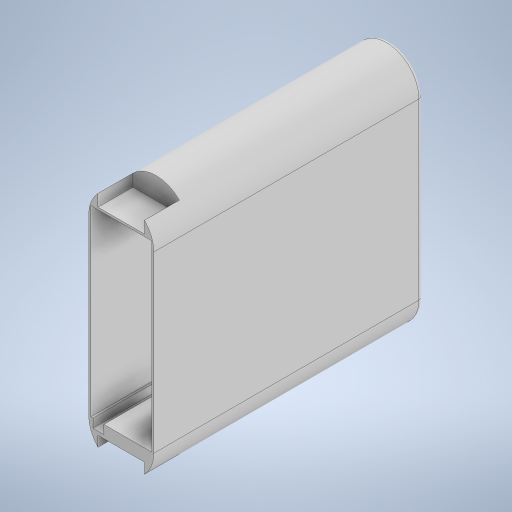
# Autodesk Inventor part: Carcasa Luis
Saved by Autodesk Inventor 2023.4 (Build 274418000, 418)
## iProperties
Created: 2024-01-25
Part Number: Carcasa Luis
Material: Genérico
Document SubType Name: Modeling
Designer: Adrián Álvarez
Density: 1 g/cm^3
Appearance: Valor por defecto
Author: Adrián Álvarez
Autodesk Inventor part; units mm, degrees
ref_plane "YZ Plane" through (0, 0, 0) normal (1, 0, 0) x (0, 1, 0)
ref_plane "XZ Plane" through (0, 0, 0) normal (0, 1, 0) x (-1, 0, 0)
ref_plane "XY Plane" through (0, 0, 0) normal (0, 0, 1) x (1, 0, 0)
sketch "Boceto1" plane through (0, 0, 0) normal (0, 0, 1) x (1, 0, 0)
  line L0 (0, 0) -> (0, 40.1) construction
  line L1 (7.5, 0) -> (7.5, 40.1)
  line L2 (-7.5, 40.1) -> (-7.5, 0)
  arc A0 (-7.5, 0) -> (7.5, 0) centre (0, 0) ccw
  arc A1 (7.5, 40.1) -> (-7.5, 40.1) centre (0, 40.1) ccw
  point P0 (0, 20.05)
  dimension "d0" = 40.1
  dimension "d1" = 15
  constraints: 8 end point, 4 point on circle, 4 tangent, 2 centre point, 1 midpoint, 1 parallel, 1 vertical
  measures "d0" distance of L0.start L0.end
  measures "d1" diameter of A1
extrude "Extrusión1" add sketch "Boceto1" along normal blind 62
sketch "Boceto2" plane through (0, 0, 62) normal (0, 0, 1) x (1, 0, 0)
  line L0 (0, 0) -> (-7, 0)
  line L1 (-7, 0) -> (-7, 40.0875)
  line L2 (-7.5, 40.1) -> (-7.5, 0) projected
  line L3 (7, 0) -> (-7, 0)
  line L4 (-7, 40.0875) -> (-7, 42.1)
  arc A0 (7.5, 40.1) -> (-7.5, 40.1) centre (0, 40.1) ccw projected
  line L5 (-7, 42.1) -> (7, 42.1)
  line L6 (7, 42.1) -> (7, 0)
  dimension "d4" = 7
  dimension "d68" = 7
  dimension "d69" = 14
  constraints: 12 end point, 2 horizontal, 1 parallel, 1 perpendicular, 1 vertical
  measures "d4" distance of L0.start L0.end
  measures "d68" distance of L3.start L0.start
  measures "d69" distance of L4.end L5.end
extrude "Extrusión2" cut sketch "Boceto2" against normal blind 61
sketch "Boceto3" plane through (0, 0, 62) normal (0, 0, 1) x (1, 0, 0)
  line L0 (-5.3571, -2.8499) -> (5.3571, -2.8499)
  line L1 (-6.5, 40.1) -> (6.5, 40.1) projected
  line L2 (-5, 42.6) -> (5, 42.6)
  line L3 (-5.3571, -2.8499) -> (-5.3571, -4.1499)
  line L4 (5.3571, -5.2489) -> (5.3571, -2.8499)
  arc A0 (7.5, 40.1) -> (-7.5, 40.1) centre (0, 40.1) ccw projected
  arc A1 (-5.3571, -5.2489) -> (5.3571, -5.2489) centre (0, 0) ccw
  line L5 (-5.3571, -4.1499) -> (-5.3571, -5.2489)
  arc A2 (-7.5, 0) -> (7.5, 0) centre (0, 0) ccw projected
  arc A3 (5.357, 45.3491) -> (-5.357, 45.3491) centre (0, 40.1) ccw
  line L6 (0, 42.6) -> (-5.357, 42.6)
  line L7 (-5.357, 42.6) -> (-5.357, 45.3491)
  line L8 (0, 42.6) -> (5.357, 42.6)
  line L9 (5.357, 42.6) -> (5.357, 45.3491)
  line L10 (0, -2.8499) -> (-5.357, -2.8499)
  point P0 (5.3571, -4.1499)
  point P1 (5, 43.9)
  dimension "d46" = 1.3
  dimension "d70" = 5.357
  dimension "d71" = 5.357
  dimension "d72" = 5.357
  constraints: 20 end point, 5 point on circle, 4 point on line, 2 centre point, 2 coincident, 2 midpoint, 2 perpendicular, 2 vertical
  measures "d46" distance of L0.start L3.end
  measures "d70" distance of L6.start L6.end
  measures "d71" distance of L6.start L8.end
  measures "d72" distance of L10.start L10.end
extrude "Extrusión3" cut sketch "Boceto3" against normal blind 8
fillet "Empalme1" radius 1 4 edges at (0, 47.6, 0) (-7.5, 20.05, 0) (0, -7.5, 0) (7.5, 20.05, 0)
sketch "Boceto5" plane through (0, 0, 62) normal (0, 0, 1) x (1, 0, 0)
  line L0 (7, 0) -> (-7, 0) projected
  line L1 (7, 0) -> (-3.5, 0)
  line L2 (5, -1) -> (-5, -1) projected
  line L3 (-3.5, -0.9) -> (-2, -0.9) construction
  arc A0 (-6.5, 0) -> (6.5, 0) centre (0, 0) ccw projected
  line L4 (-6.5, 0) -> (-3.5, 0)
  line L5 (-6.5, 0) -> (-6.5, -2)
  line L6 (-6.5, -2) -> (-5, -2)
  line L7 (-5, -2) -> (-4, -2)
  line L8 (-4, -2) -> (-4, 0)
  line L9 (7, 0) -> (-7, 0) projected
  dimension "d49" = 2
  dimension "d51" = 1
  constraints: 14 end point, 2 horizontal, 2 point on line, 1 collinear, 1 parallel, 1 perpendicular, 1 tangent, 1 vertical
  measures "d49" distance of L4.start L5.end
  measures "d51" distance of L6.end L7.end
extrude "Extrusión5" cut sketch "Boceto5" against normal blind 60 contours L6 L5 A0 | A0 L0 L8 L7 L6 picked at (-5.1549, -1.2255)
sketch "Boceto6" plane through (0, 0, 0) normal (0, 0, -1) x (-1, 0, 0)
  line L0 (-7, 0) -> (7, 0) projected
  line L1 (3.5, 0) -> (3.5, 6.5)
  line L2 (6.5, 40.1) -> (-6.5, 40.1) projected
  line L3 (-0.5, 0) -> (3.5, 0)
  line L4 (7, 0) -> (7, 42.1) projected
  line L5 (6.5, 40.1) -> (6.5, 0) projected
  line L6 (4.5, 6.5) -> (4.5, 15.5)
  line L7 (4.5, 15.5) -> (0.5, 15.5)
  line L8 (0.5, 15.5) -> (0.5, 6.5)
  line L9 (-0.5, 0) -> (0.5, 0)
  line L10 (-7, 0) -> (7, 0) projected
  line L11 (0.5, 0) -> (0.5, 6.5)
  line L12 (4.5, 6.5) -> (0.5, 6.5)
  point P0 (0, 0)
  point P1 (7, 42.1)
  dimension "d44" = 9
  dimension "d60" = 1
  constraints: 16 end point, 2 horizontal, 2 perpendicular, 2 point on line, 1 vertical, 1 other
  measures "d44" distance of L6.start L6.end
  measures "d60" distance of L3.start L9.end
extrude "Extrusión6" cut sketch "Boceto6" against normal through all contours L8 L7 L6 L12
sketch "Boceto7" plane through (-7.5, 0, 62) normal (-1, 0, 0) x (0, 0, 1)
  line L0 (-45, 36.8) -> (-45, 38.6)
  line L1 (-45, 38.6) -> (-51, 38.6)
  line L2 (-51, 38.6) -> (-51, 36.8)
  line L3 (-51, 36.8) -> (-45, 36.8)
  point P0 (-62, 0)
  dimension "d74" = 6
  constraints: 8 end point, 2 perpendicular, 1 horizontal
  measures "d74" distance of L0.end L1.end
extrude "Extrusión7" cut sketch "Boceto7" against normal blind 3
sketch "Boceto8" plane through (0, 0, 0) normal (0, 0, -1) x (-1, 0, 0)
  line L0 (0.5, 6.5) -> (0.5, 15.5) projected
  line L1 (4.5, 15.5) -> (4.5, 6.5) projected
  line L2 (0.5, 15.5) -> (4.5, 15.5)
  line L3 (4.5, 15.5) -> (4.5, 6.5)
  line L4 (4.5, 6.5) -> (0.5, 6.5)
  line L5 (0.5, 6.5) -> (0.5, 15.5)
  line L6 (5.5, 16.5) -> (-0.5, 16.5)
  line L7 (-0.5, 16.5) -> (-0.5, 5.5)
  line L8 (-0.5, 5.5) -> (5.5, 5.5)
  line L9 (5.5, 5.5) -> (5.5, 16.5)
  point P0 (0, 0)
  dimension "d61" = 1
  constraints: 16 end point, 4 parallel, 2 perpendicular, 1 horizontal, 3 other
  measures "d61" distance between parallel lines of L2 L6
extrude "Extrusión8" cut sketch "Boceto8" against normal blind 0.5 contours L0 L2 L1 L4 | L9 L8 L7 L6
sketch "Boceto9" plane through (-7.5, 0, 62) normal (-1, 0, 0) x (0, 0, 1)
  point P0 (-62, 0)
